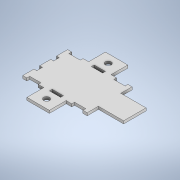
# Autodesk Inventor part: v4_Burrow_Base_Detachable_EXT
Saved by Autodesk Inventor 2020.4 (Build 244396010, 396A)
## iProperties
Created: 2021-09-30
Part Number: v4_Burrow_Base_Detachable_EXT
Material: Generic
Document SubType Name: Sheet Metal
Designer: YUSTE
Density: 1 g/cm^3
Sheet Metal Rule: Default
Appearance: Default
Author: YUSTE
Autodesk Inventor part; units mm, degrees
ref_plane "YZ Plane" through (0, 0, 0) normal (1, 0, 0) x (0, 1, 0)
ref_plane "XZ Plane" through (0, 0, 0) normal (0, 1, 0) x (-1, 0, 0)
ref_plane "XY Plane" through (0, 0, 0) normal (0, 0, 1) x (1, 0, 0)
sketch "Sketch1" plane through (0, 0, 0) normal (0, 1, 0) x (-1, 0, 0)
  line L0 (0, 0) -> (101.6, 0)
  line L1 (101.6, 0) -> (101.6, 50.8)
  line L2 (101.6, 50.8) -> (0, 50.8)
  line L3 (0, 50.8) -> (0, 0)
  line L4 (101.6, 0) -> (28.575, 0)
  line L5 (28.575, 0) -> (28.575, 50.8)
  line L6 (28.575, 50.8) -> (101.6, 50.8)
  line L7 (101.6, 50.8) -> (101.6, 0)
  line L8 (28.575, 0) -> (0, 0)
  line L9 (0, 0) -> (0, 12.7)
  line L10 (0, 12.7) -> (28.575, 12.7)
  line L11 (28.575, 12.7) -> (28.575, 0)
  line L12 (28.575, 50.8) -> (0, 50.8)
  line L13 (0, 50.8) -> (0, 38.1)
  line L14 (0, 38.1) -> (28.575, 38.1)
  line L15 (28.575, 38.1) -> (28.575, 50.8)
  line L16 (96.8375, 0) -> (84.1375, 0)
  line L17 (84.1375, 0) -> (84.1375, 3.175)
  line L18 (84.1375, 3.175) -> (96.8375, 3.175)
  line L19 (96.8375, 3.175) -> (96.8375, 0)
  line L20 (71.4375, 0) -> (58.7375, 0)
  line L21 (58.7375, 0) -> (58.7375, 3.175)
  line L22 (58.7375, 3.175) -> (71.4375, 3.175)
  line L23 (71.4375, 3.175) -> (71.4375, 0)
  line L24 (46.0375, 0) -> (33.3375, 0)
  line L25 (33.3375, 0) -> (33.3375, 3.175)
  line L26 (33.3375, 3.175) -> (46.0375, 3.175)
  line L27 (46.0375, 3.175) -> (46.0375, 0)
  line L28 (96.8375, 50.8) -> (84.1375, 50.8)
  line L29 (84.1375, 50.8) -> (84.1375, 47.625)
  line L30 (84.1375, 47.625) -> (96.8375, 47.625)
  line L31 (96.8375, 47.625) -> (96.8375, 50.8)
  line L32 (71.4375, 50.8) -> (58.7375, 50.8)
  line L33 (58.7375, 50.8) -> (58.7375, 47.625)
  line L34 (58.7375, 47.625) -> (71.4375, 47.625)
  line L35 (71.4375, 47.625) -> (71.4375, 50.8)
  line L36 (101.6, 38.1) -> (98.425, 38.1)
  line L37 (98.425, 38.1) -> (98.425, 31.75)
  line L38 (98.425, 31.75) -> (101.6, 31.75)
  line L39 (101.6, 31.75) -> (101.6, 38.1)
  line L40 (101.6, 19.05) -> (98.425, 19.05)
  line L41 (98.425, 19.05) -> (98.425, 12.7)
  line L42 (98.425, 12.7) -> (101.6, 12.7)
  line L43 (101.6, 12.7) -> (101.6, 19.05)
  line L44 (46.0375, 50.8) -> (46.0375, 47.625)
  line L45 (46.0375, 47.625) -> (33.3375, 47.625)
  line L46 (33.3375, 47.625) -> (33.3375, 50.8)
  line L47 (33.3375, 50.8) -> (46.0375, 50.8)
  line L48 (52.3875, 0) -> (77.7875, 0)
  line L49 (77.7875, 0) -> (77.7875, -19.05)
  line L50 (77.7875, -19.05) -> (52.3875, -19.05)
  line L51 (52.3875, -19.05) -> (52.3875, 0)
  line L52 (52.3875, 50.8) -> (52.3875, 69.85)
  line L53 (52.3875, 69.85) -> (77.7875, 69.85)
  line L54 (77.7875, 69.85) -> (77.7875, 50.8)
  line L55 (77.7875, 50.8) -> (52.3875, 50.8)
  circle A0 centre (65.0875, -9.525) radius 3.302
  circle A1 centre (65.0875, 60.325) radius 3.302
  point P0 (96.8375, 0)
  point P1 (96.8375, 50.8)
  point P2 (84.1375, 50.8)
  point P3 (71.4375, 50.8)
  point P4 (58.7375, 50.8)
  point P5 (46.0375, 50.8)
  point P6 (33.3375, 50.8)
  point P7 (33.3375, 0)
  point P8 (46.0375, 0)
  point P9 (58.7375, 0)
  point P10 (71.4375, 0)
  point P11 (84.1375, 0)
  dimension "d56" = 101.6
  dimension "d57" = 50.8
  dimension "d58" = 73.025
  dimension "d59" = 50.8
  dimension "d60" = 12.7
  dimension "d61" = 12.7
  dimension "d62" = 12.7
  dimension "d63" = 3.175
  dimension "d64" = 12.7
  dimension "d65" = 3.175
  dimension "d66" = 12.7
  dimension "d67" = 4.7625
  dimension "d68" = 12.7
  dimension "d69" = 3.175
  dimension "d70" = 12.7
  dimension "d71" = 12.7
  dimension "d72" = 3.175
  dimension "d73" = 12.7
  dimension "d74" = 3.175
  dimension "d77" = 4.7625
  dimension "d78" = 12.7
  dimension "d79" = 3.175
  dimension "d80" = 6.35
  dimension "d81" = 12.7
  dimension "d82" = 3.175
  dimension "d83" = 6.35
  dimension "d84" = 12.7
  dimension "d86" = 44.45
  dimension "d89" = 3.175
  dimension "d90" = 12.7
  dimension "d91" = 12.7
  dimension "d94" = 25.4
  dimension "d96" = 23.8125
  dimension "d97" = 23.8125
  dimension "d99" = 25.4
  dimension "d116" = 6.604
  dimension "d117" = 9.525
  dimension "d118" = 6.604
  dimension "d119" = 9.525
  dimension "d122" = 9.525
  dimension "d123" = 9.525
  measures "d56" distance of L0.start L0.end
  measures "d57" distance of L1.end L0.end
  measures "d58" distance of L0.end L5.start
  measures "d59" distance of L5.start L5.end
  measures "d60" distance of L0.start L9.end
  measures "d61" distance of L13.end L2.end
  measures "d62" distance of L16.start L16.end
  measures "d63" distance of L16.end L17.end
  measures "d64" distance of L20.start L20.end
  measures "d65" distance of L20.end L21.end
  measures "d66" distance between parallel lines of L17 L23
  measures "d67" distance between parallel lines of L1 L19
  measures "d68" distance of L24.start L24.end
  measures "d69" distance of L24.end L25.end
  measures "d70" distance between parallel lines of L27 L21
  measures "d71" distance of L28.start L28.end
  measures "d72" distance of L29.end L28.end
  measures "d73" distance of L32.start L32.end
  measures "d74" distance of L33.end L32.end
  measures "d77" distance between parallel lines of L1 L31
  measures "d78" distance between parallel lines of L35 L29
  measures "d79" distance of L36.start L36.end
  measures "d80" distance of L37.end L36.end
  measures "d81" distance between parallel lines of L2 L36
  measures "d82" distance of L40.start L40.end
  measures "d83" distance of L41.end L40.end
  measures "d84" distance between parallel lines of L0 L42
  measures "d86" distance between parallel lines of L30 L18
  measures "d89" distance of L44.start L44.end
  measures "d90" distance of L44.end L45.end
  measures "d91" distance between parallel lines of L44 L33
  measures "d94" distance of L48.start L48.end
  measures "d96" distance between parallel lines of L1 L49
  measures "d97" distance between parallel lines of L11 L51
  measures "d99" distance of L52.end L53.end
  measures "d116" diameter of A0
  measures "d117" distance from line of L20 A0.centre
  measures "d118" diameter of A1
  measures "d119" distance from line of L32 A1.centre
  measures "d122" distance from line of L50 A0.centre
  measures "d123" distance from line of L53 A1.centre
extrude "Plate4" add sketch "Sketch1" along normal blind 3.048 contours L5 L2 L46 L45 L44 L33 L34 L35 L29 L30 L31 L1 L36 L37 L38 L40 L41 L42 L0 L19 L18 L17 L23 L22 L21 L27 L26 L25 | L3 L14 L5 L10 | L0 L49 L50 L51 | L52 L53 L54 L2
equation "\"d127\" = Thickness"
equation "\"BendRadius\" = Thickness"
equation "\"BendReliefWidth\" = Thickness"
equation "\"BendReliefDepth\" = 0.5 * Thickness"
equation "\"CornerReliefSize\" = 4 * Thickness"
equation "\"MinimumRemnant\" = 2 * Thickness"
equation "\"TransitionRadius\" = BendRadius"
equation "\"JacobiRadiusSize\" = BendRadius"
equation "\"GapSize\" = Thickness"
equation "\"Thickness\" = 3.048"
body "Solid8"
